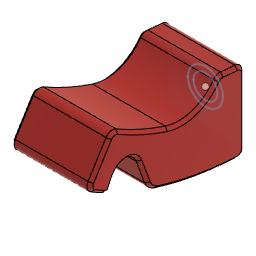
latch_shuttle (Autodesk Fusion 360 design; units mm, degrees)
Autodesk Fusion 360 part; units mm, degrees
sketch "Sketch1" plane through (0, 0, 0) normal (1, 0, 0) x (0, 1, 0) in component "latch_shuttle"
  arc A0 (-8.3077, 5.5575) -> (-1.6746, 2.5672) centre (9.4182, 36.0259) ccw
  arc A1 (-8.3077, 5.5575) -> (-9.6608, 5.2196) centre (-8.8106, 4.6931) ccw
  line L0 (-12.0836, 1.3076) -> (-9.6608, 5.2196)
  arc A2 (-12.0836, 1.3076) -> (-11.739, -0.0818) centre (-11.2334, 0.781) ccw
  arc A3 (-11.739, -0.0818) -> (-10.3245, -0.8742) centre (9.4182, 36.0259) ccw
  arc A4 (-10.3245, -0.8742) -> (-9.5002, -0.6041) centre (-10.0414, -0.3452) ccw
  line L1 (-9.5002, -0.6041) -> (-8.9235, 0.6015)
  arc A5 (-5.6086, 0.4414) -> (-8.9235, 0.6015) centre (-7.2997, -0.1753) ccw
  line L2 (-5.6086, 0.4414) -> (-4.4802, -2.6531)
  arc A6 (-4.4802, -2.6531) -> (-3.2044, -3.8747) centre (-2.6012, -1.9679) ccw
  arc A7 (-3.2044, -3.8747) -> (7.5742, -5.7831) centre (9.4182, 36.0259) ccw
  arc A8 (7.5742, -5.7831) -> (8.6182, -4.784) centre (7.6182, -4.784) ccw
  line L3 (8.6182, 3.9982) -> (8.6182, -4.784)
  arc A9 (8.6182, 3.9982) -> (7.6743, 4.9966) centre (7.6182, 3.9982) ccw
  arc A10 (5.7512, 5.1647) -> (7.6743, 4.9966) centre (9.4182, 36.0259) ccw
  arc A11 (5.7512, 5.1647) -> (4.8102, 4.7397) centre (5.6332, 4.1717) ccw
  arc A12 (-1.6746, 2.5672) -> (4.8102, 4.7397) centre (0.1191, 7.9776) ccw
extrude "Extrude1" add sketch "Sketch1" along normal mid plane 10.6 in component "latch_shuttle"
chamfer "Chamfer1" distance 0.4 angle 45 34 edges at (5.3, -5.0685, 3.8907) (5.3, -9.0529, 5.6633) (5.3, -10.8722, 3.2636) (5.3, -12.204, 0.5403) (5.3, -11.0356, -0.4848) (5.3, -9.8546, -0.9153) (5.3, -9.2118, -0.0013) (5.3, -7.2129, 1.6226) (5.3, -5.0444, -1.1058) (5.3, -3.9845, -3.4124) (5.3, 2.1222, -5.1828) (5.3, 8.3096, -5.5066) (5.3, 8.6182, -0.3929) (5.3, 8.3449, 4.6851) (5.3, 6.7115, 5.0657) (5.3, 5.2216, 5.0831) (5.3, 1.9298, 2.5728) (-5.3, 8.6182, -0.3929) (-5.3, 8.3096, -5.5066) (-5.3, 2.1222, -5.1828) (-5.3, -3.9845, -3.4124) (-5.3, -5.0444, -1.1058) (-5.3, -7.2129, 1.6226) (-5.3, -9.2118, -0.0013) (-5.3, -9.8546, -0.9153) (-5.3, -11.0356, -0.4848) (-5.3, -12.204, 0.5403) (-5.3, -10.8722, 3.2636) (-5.3, -9.0529, 5.6633) (-5.3, -5.0685, 3.8907) (-5.3, 1.9298, 2.5728) (-5.3, 5.2216, 5.0831) (-5.3, 6.7115, 5.0657) (-5.3, 8.3449, 4.6851) in component "latch_shuttle"
sketch "Sketch2" plane through (0, 8.6182, 0) normal (0, 1, 0) x (-1, 0, 0) in component "latch_shuttle"
  line L0 (4.9, -4.784) -> (4.9, 3.9982)
  line L1 (4.9, 3.9982) -> (-4.9, 3.9982)
  line L2 (-4.9, 3.9982) -> (-4.9, -4.784)
  line L3 (-4.9, -4.784) -> (4.9, -4.784)
  circle A0 centre (0, -0.4177) radius 1.6
  circle A1 centre (0, -0.4177) radius 2.35
extrude "Extrude2" cut sketch "Sketch2" against normal blind 4.2 contours A0 | A1 in component "latch_shuttle"
extrude "Extrude3" cut sketch "Sketch2" against normal blind 12 contours A0 in component "latch_shuttle"
component "latch_shuttle" placed x (1, 0, 0) y (0, 1, 0) z (0, 0, 1) at (0, 0, 0)
